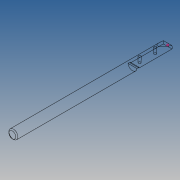
# Autodesk Inventor part: J007626
Saved by Autodesk Inventor 2018.3 (Build 223284000, 284)
## iProperties
Created: 2017-02-24
Material: ALUMINUM, 6061-T651
Vendor: HHMI: JRC - ID&F
Document SubType Name: Modeling
Designer: ARNOLDJ
Density: 2.7 g/cm^3
Appearance: Metal-AL-6061 (Machined)
Description: PTR RECORDING POST 1/4" DIA EXTENDED
Project: COMMON
Part Number: J007626
RuleStatus: InUse
AfterDocSave0: file://Part Number Cleaner
LAB/DEPT: APIG (SHARED RESOURCE)
REQUESTING SCIENTIST: COMMON
SURFACE ROUGHNESS: 63 Ra
DESIGN DEPARTMENT: HHMI: JRC - ID&F
SPECIAL FINISH: NONE
ALTERED ITEM PART NUMBER: N/A
ALTERED ITEM VENDOR: N/A
ALTERED ITEM DESCRIPTION: N/A
Author: ARNOLDJ
Revision Number: -
Autodesk Inventor part; units mm, degrees
ref_plane "YZ Plane" through (0, 0, 0) normal (1, 0, 0) x (0, 1, 0)
ref_plane "XZ Plane" through (0, 0, 0) normal (0, 1, 0) x (-1, 0, 0)
ref_plane "XY Plane" through (0, 0, 0) normal (0, 0, 1) x (1, 0, 0)
sketch "Sketch1" plane through (0, 0, 0) normal (0, 0, 1) x (1, 0, 0)
  point P0 (0, 0)
sketch "Sketch2" plane through (0, 0, 0) normal (0, 0, 1) x (1, 0, 0)
  line L0 (0, 4.445) -> (0, -4.445) projected
  line L1 (-4.445, 0) -> (4.445, 0) projected
  circle A0 centre (0, 0) radius 3.175
  dimension "d0" = 6.35
  constraints: 1 centre point, 1 coincident
  measures "d0" diameter of A0
extrude "Extrusion1" add sketch "Sketch2" along normal blind 109.22
sketch "Sketch3" plane through (0, 0, 0) normal (1, 0, 0) x (0, 1, 0)
  line L0 (0, 29.718) -> (0, -4.953) projected
  line L1 (-4.445, 0) -> (4.445, 0) projected
  line L2 (-3.175, 0) -> (3.175, 0) projected
  line L3 (-3.175, 0) -> (-0.7874, 0)
  line L4 (-0.7874, 0) -> (-0.7874, 24.765)
  line L5 (-0.7874, 24.765) -> (-3.175, 24.765)
  line L6 (-3.175, 24.765) -> (-3.175, 0)
  line L7 (-0.7874, 24.765) -> (-0.2794, 24.765)
  line L8 (-0.2794, 24.765) -> (-0.2794, 23.241)
  line L9 (-0.2794, 23.241) -> (-0.7874, 23.241)
  line L10 (-0.7874, 23.241) -> (-0.7874, 24.765)
  point P0 (0, 0)
  dimension "d3" = 24.765
  dimension "d4" = 0.508
  dimension "d5" = 1.524
  dimension "d6" = 3.9624
  constraints: 16 end point, 4 parallel, 2 horizontal, 2 perpendicular
  measures "d3" distance of L3.end L4.end
  measures "d4" distance of L4.end L7.end
  measures "d5" distance of L7.end L8.end
  measures "d6" distance from line of L4 L2.end
extrude "Extrusion2" cut sketch "Sketch3" along normal mid plane 25.4
sketch "Sketch4" plane through (0, -0.7874, -0.635) normal (0, 1, 0) x (-1, 0, 0)
  line L0 (-3.0758, 0.635) -> (3.0758, 0.635) projected
  line L1 (0, -21.209) -> (0, 131.699) projected
  line L2 (3.1627, 25.4) -> (-3.1627, 25.4) projected
  point P0 (0, 0.635)
  point P1 (0, 9.398)
  point P2 (3.1627, 25.4)
  point P3 (-3.1627, 25.4)
  point P4 (0, 20.398)
  dimension "d13" = 16.002
  dimension "d14" = 11
  constraints: 2 point on line
  measures "d13" distance from line of L2 point (0, 9.398)
  measures "d14" distance of point (0, 9.398) point (0, 20.398)
hole "Hole1" at (0, -0.7874, 8.763) at (0, -0.7874, 19.763) direction (0, 1, 0) diameter 1.5748 end through all
chamfer "Chamfer1" distance 0.762 angle 45 1 edges at (-3.175, 0, 109.22)
sketch "Sketch5" plane through (0, 0, 0) normal (1, 0, 0) x (0, 1, 0)
  line L0 (3.175, 0) -> (3.175, 108.458) projected
  line L1 (-1.5799, 0) -> (3.9675, 0) projected
  line L2 (3.175, 0) -> (3.175, 7.2044)
  line L3 (3.175, 7.2044) -> (1.2446, 0)
  line L4 (-0.7874, 0) -> (3.175, 0) projected
  line L5 (1.2446, 0) -> (3.175, 0)
  line L6 (-0.7874, 0) -> (-0.7874, 23.241) projected
  point P0 (0, 0)
  dimension "d22" = 1.9304
  dimension "d26" = 2.032
  dimension "d27" = 15
  constraints: 6 end point, 2 point on line, 1 horizontal
  measures "d22" distance from line of L0 L3.end
  measures "d26" distance from line of L3.end L6
  measures "d27" angle of L0 L3
extrude "Extrusion3" cut sketch "Sketch5" along normal mid plane 25.4
body "Solid1"
